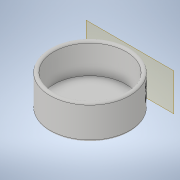
# Autodesk Inventor part: LargeFinderObjectiveCover
Saved by Autodesk Inventor 2021.1 (Build 251245000, 245)
## iProperties
Created: 2018-09-01
Part Number: LargeFinderObjectiveCover
Material: Generic
Document SubType Name: Modeling
Designer: steele
Density: 1 g/cm^3
Appearance: Default
Author: steele
Autodesk Inventor part; units mm, degrees
ref_plane "YZ Plane" through (0, 0, 0) normal (1, 0, 0) x (0, 1, 0)
ref_plane "XZ Plane" through (0, 0, 0) normal (0, 1, 0) x (-1, 0, 0)
sketch "Sketch1" plane through (0, 0, 0) normal (0, 1, 0) x (-1, 0, 0)
  circle A0 centre (0, 0) radius 33.655
  dimension "d0" = 67.31
  constraints: 1 centre point, 1 coincident
  measures "d0" diameter of A0
extrude "Extrusion1" add sketch "Sketch1" along normal blind 3.175
sketch "Sketch2" plane through (0, 3.175, 0) normal (0, 1, 0) x (1, 0, 0)
  circle A0 centre (0, 0) radius 33.655
  circle A1 centre (0, 0) radius 30.48
  dimension "d4" = 60.96
  dimension "d5" = 67.31
  constraints: 2 centre point, 1 coincident
  measures "d4" diameter of A1
  measures "d5" diameter of A0
extrude "Extrusion3" add sketch "Sketch2" along normal blind 25.4
ref_plane "Work Plane1" through (0, 0, -33.655) normal (0, 0, 1) x (1, 0, 0)
sketch "Sketch5" plane through (0, 0, -33.655) normal (0, 0, 1) x (1, 0, 0)
  line L0 (-33.655, 0) -> (-33.655, 28.575) projected
  line L1 (33.655, 0) -> (33.655, 28.575) projected
  line L2 (33.655, 14.2875) -> (-33.655, 14.2875) construction
  line L3 (2.2158, 14.2875) -> (0.248, 14.2875)
  line L4 (0.248, 14.2875) -> (0.248, 13.7688)
  line L5 (0.248, 13.7688) -> (0.8944, 13.7688)
  line L6 (0.8944, 13.7688) -> (0.8944, 9.7262)
  line L7 (0.8944, 9.7262) -> (0.248, 9.7262)
  line L8 (0.248, 9.7262) -> (0.248, 9.2075)
  line L9 (0.248, 9.2075) -> (2.2158, 9.2075)
  line L10 (2.2158, 9.2075) -> (2.2158, 9.7262)
  line L11 (2.2158, 9.7262) -> (1.5695, 9.7262)
  line L12 (1.5695, 9.7262) -> (1.5695, 13.7688)
  line L13 (1.5695, 13.7688) -> (2.2158, 13.7688)
  line L14 (2.2158, 13.7688) -> (2.2158, 14.2875)
  spline S0 degree 2 poles (7.057, 11.7516) (7.057, 12.4473) (6.4931, 13.5671) (6.0196, 13.8799) knots 0 0 0 1 2 2 2
  spline S1 degree 2 poles (6.0196, 13.8799) (5.6327, 14.1228) (4.8381, 14.2875) (4.2206, 14.2875) knots 0 0 0 1 2 2 2
  line L15 (4.2206, 14.2875) -> (3.0515, 14.2875)
  line L16 (3.0515, 14.2875) -> (3.0515, 9.2075)
  line L17 (3.0515, 9.2075) -> (4.2083, 9.2075)
  spline S2 degree 2 poles (4.2083, 9.2075) (4.9246, 9.2075) (5.7397, 9.4216) (6.0279, 9.6109) knots 0 0 0 1 2 2 2
  spline S3 degree 2 poles (6.0279, 9.6109) (6.5178, 9.9362) (7.057, 11.0106) (7.057, 11.7516) knots 0 0 0 1 2 2 2
  spline S4 degree 2 poles (6.3531, 11.7434) (6.3531, 11.1588) (5.9661, 10.3314) (5.5833, 10.0967) knots 0 0 0 1 2 2 2
  spline S5 degree 2 poles (5.5833, 10.0967) (5.3116, 9.9362) (4.6982, 9.7921) (4.2412, 9.7921) knots 0 0 0 1 2 2 2
  line L18 (4.2412, 9.7921) -> (3.7266, 9.7921)
  line L19 (3.7266, 9.7921) -> (3.7266, 13.7029)
  line L20 (3.7266, 13.7029) -> (4.2412, 13.7029)
  spline S6 degree 2 poles (4.2412, 13.7029) (4.6899, 13.7029) (5.3692, 13.5588) (5.645, 13.3654) knots 0 0 0 1 2 2 2
  spline S7 degree 2 poles (5.645, 13.3654) (5.9991, 13.1266) (6.3531, 12.3362) (6.3531, 11.7434) knots 0 0 0 1 2 2 2
  line L21 (13.2815, 14.2875) -> (12.4664, 14.2875)
  line L22 (12.4664, 14.2875) -> (12.4664, 13.316)
  line L23 (12.4664, 13.316) -> (13.2815, 13.316)
  line L24 (13.2815, 13.316) -> (13.2815, 14.2875)
  line L25 (13.2815, 11.447) -> (12.4664, 11.447)
  line L26 (12.4664, 11.447) -> (12.4664, 10.4754)
  line L27 (12.4664, 10.4754) -> (13.2815, 10.4754)
  line L28 (13.2815, 10.4754) -> (13.2815, 11.447)
  line L29 (19.7941, 14.2875) -> (16.6613, 14.2875)
  line L30 (16.6613, 14.2875) -> (16.6613, 13.5671)
  spline S8 degree 2 poles (16.6613, 13.5671) (16.9989, 13.2501) (17.5999, 12.6614) (17.8881, 12.3444) knots 0 0 0 1 2 2 2
  spline S9 degree 2 poles (17.8881, 12.3444) (18.4685, 11.7063) (18.8925, 10.9406) (18.8925, 10.5331) knots 0 0 0 1 2 2 2
  spline S10 degree 2 poles (18.8925, 10.5331) (18.8925, 10.319) (18.7608, 9.9979) (18.6414, 9.895) knots 0 0 0 1 2 2 2
  spline S11 degree 2 poles (18.6414, 9.895) (18.522, 9.7921) (18.2092, 9.6892) (18.0198, 9.6892) knots 0 0 0 1 2 2 2
  spline S12 degree 2 poles (18.0198, 9.6892) (17.8387, 9.6892) (17.4682, 9.7797) (17.2994, 9.8497) knots 0 0 0 1 2 2 2
  spline S13 degree 2 poles (17.2994, 9.8497) (17.1553, 9.9073) (16.8877, 10.072) (16.8054, 10.1296) knots 0 0 0 1 2 2 2
  line L31 (16.8054, 10.1296) -> (16.7683, 10.1296)
  line L32 (16.7683, 10.1296) -> (16.7683, 9.4051)
  spline S14 degree 2 poles (16.7683, 9.4051) (16.9783, 9.3022) (17.7316, 9.1005) (18.0692, 9.1005) knots 0 0 0 1 2 2 2
  spline S15 degree 2 poles (18.0692, 9.1005) (18.7814, 9.1005) (19.5841, 9.8538) (19.5841, 10.496) knots 0 0 0 1 2 2 2
  spline S16 degree 2 poles (19.5841, 10.496) (19.5841, 10.7965) (19.4442, 11.2988) (19.3207, 11.5128) knots 0 0 0 1 2 2 2
  spline S17 degree 2 poles (19.3207, 11.5128) (19.1972, 11.7351) (18.839, 12.1715) (18.6414, 12.3815) knots 0 0 0 1 2 2 2
  spline S18 degree 2 poles (18.6414, 12.3815) (18.3203, 12.7314) (17.534, 13.4806) (17.2994, 13.6988) knots 0 0 0 1 2 2 2
  line L33 (17.2994, 13.6988) -> (19.7941, 13.6988)
  line L34 (19.7941, 13.6988) -> (19.7941, 14.2875)
  line L35 (21.5643, 14.2875) -> (20.7492, 14.2875)
  line L36 (20.7492, 14.2875) -> (20.7492, 13.316)
  line L37 (20.7492, 13.316) -> (21.5643, 13.316)
  line L38 (21.5643, 13.316) -> (21.5643, 14.2875)
  line L39 (25.858, 12.542) -> (25.2528, 12.542)
  line L40 (25.2528, 12.542) -> (25.2528, 14.2875)
  line L41 (25.2528, 14.2875) -> (24.5983, 14.2875)
  line L42 (24.5983, 14.2875) -> (24.5983, 12.542)
  line L43 (24.5983, 12.542) -> (22.3547, 12.542)
  line L44 (22.3547, 12.542) -> (22.3547, 11.8257)
  line L45 (22.3547, 11.8257) -> (24.6271, 9.2075)
  line L46 (24.6271, 9.2075) -> (25.2528, 9.2075)
  line L47 (25.2528, 9.2075) -> (25.2528, 11.9945)
  line L48 (25.2528, 11.9945) -> (25.858, 11.9945)
  line L49 (25.858, 11.9945) -> (25.858, 12.542)
  line L50 (24.5983, 11.9945) -> (24.5983, 10.0103)
  line L51 (24.5983, 10.0103) -> (22.8898, 11.9945)
  line L52 (22.8898, 11.9945) -> (24.5983, 11.9945)
  spline S19 degree 2 poles (29.563, 11.7475) (29.563, 13.1142) (28.7685, 14.3945) (27.941, 14.3945) knots 0 0 0 1 2 2 2
  spline S20 degree 2 poles (27.941, 14.3945) (27.1012, 14.3945) (26.3149, 13.0895) (26.3149, 11.7516) knots 0 0 0 1 2 2 2
  spline S21 degree 2 poles (26.3149, 11.7516) (26.3149, 10.3766) (27.1095, 9.1046) (27.941, 9.1046) knots 0 0 0 1 2 2 2
  spline S22 degree 2 poles (27.941, 9.1046) (28.7767, 9.1046) (29.563, 10.4219) (29.563, 11.7475) knots 0 0 0 1 2 2 2
  spline S23 degree 2 poles (28.6903, 13.2954) (28.7891, 13.0443) (28.8714, 12.2703) (28.8714, 11.7475) knots 0 0 0 1 2 2 2
  spline S24 degree 2 poles (28.8714, 11.7475) (28.8714, 11.2247) (28.7891, 10.4549) (28.6862, 10.1955) knots 0 0 0 1 2 2 2
  spline S25 degree 2 poles (28.6862, 10.1955) (28.5832, 9.9362) (28.2251, 9.6686) (27.941, 9.6686) knots 0 0 0 1 2 2 2
  spline S26 degree 2 poles (27.941, 9.6686) (27.657, 9.6686) (27.2906, 9.9362) (27.1836, 10.2037) knots 0 0 0 1 2 2 2
  spline S27 degree 2 poles (27.1836, 10.2037) (27.0806, 10.4631) (27.0065, 11.2535) (27.0065, 11.7516) knots 0 0 0 1 2 2 2
  spline S28 degree 2 poles (27.0065, 11.7516) (27.0065, 12.2868) (27.0724, 13.0031) (27.1794, 13.283) knots 0 0 0 1 2 2 2
  spline S29 degree 2 poles (27.1794, 13.283) (27.2782, 13.5465) (27.6446, 13.8305) (27.941, 13.8305) knots 0 0 0 1 2 2 2
  spline S30 degree 2 poles (27.941, 13.8305) (28.221, 13.8305) (28.5873, 13.563) (28.6903, 13.2954) knots 0 0 0 1 2 2 2
  spline S31 degree 2 poles (33.3751, 11.7475) (33.3751, 13.1142) (32.5805, 14.3945) (31.7531, 14.3945) knots 0 0 0 1 2 2 2
  spline S32 degree 2 poles (31.7531, 14.3945) (30.9133, 14.3945) (30.127, 13.0895) (30.127, 11.7516) knots 0 0 0 1 2 2 2
  spline S33 degree 2 poles (30.127, 11.7516) (30.127, 10.3766) (30.9215, 9.1046) (31.7531, 9.1046) knots 0 0 0 1 2 2 2
  spline S34 degree 2 poles (31.7531, 9.1046) (32.5888, 9.1046) (33.3751, 10.4219) (33.3751, 11.7475) knots 0 0 0 1 2 2 2
  spline S35 degree 2 poles (32.5023, 13.2954) (32.6011, 13.0443) (32.6835, 12.2703) (32.6835, 11.7475) knots 0 0 0 1 2 2 2
  spline S36 degree 2 poles (32.6835, 11.7475) (32.6835, 11.2247) (32.6011, 10.4549) (32.4982, 10.1955) knots 0 0 0 1 2 2 2
  spline S37 degree 2 poles (32.4982, 10.1955) (32.3953, 9.9362) (32.0371, 9.6686) (31.7531, 9.6686) knots 0 0 0 1 2 2 2
  spline S38 degree 2 poles (31.7531, 9.6686) (31.469, 9.6686) (31.1026, 9.9362) (30.9956, 10.2037) knots 0 0 0 1 2 2 2
  spline S39 degree 2 poles (30.9956, 10.2037) (30.8927, 10.4631) (30.8186, 11.2535) (30.8186, 11.7516) knots 0 0 0 1 2 2 2
  spline S40 degree 2 poles (30.8186, 11.7516) (30.8186, 12.2868) (30.8845, 13.0031) (30.9915, 13.283) knots 0 0 0 1 2 2 2
  spline S41 degree 2 poles (30.9915, 13.283) (31.0903, 13.5465) (31.4567, 13.8305) (31.7531, 13.8305) knots 0 0 0 1 2 2 2
  spline S42 degree 2 poles (31.7531, 13.8305) (32.033, 13.8305) (32.3994, 13.563) (32.5023, 13.2954) knots 0 0 0 1 2 2 2
  spline S43 degree 2 poles (3.8831, 18.1769) (4.1712, 18.5144) (4.4923, 19.5024) (4.4923, 20.1364) knots 0 0 0 1 2 2 2
  spline S44 degree 2 poles (4.4923, 20.1364) (4.4923, 20.7539) (4.1795, 21.7543) (3.8831, 22.0918) knots 0 0 0 1 2 2 2
  spline S45 degree 2 poles (3.8831, 22.0918) (3.5702, 22.4459) (2.7427, 22.7834) (2.2446, 22.7834) knots 0 0 0 1 2 2 2
  spline S46 degree 2 poles (2.2446, 22.7834) (1.73, 22.7834) (0.9067, 22.4335) (0.6062, 22.0918) knots 0 0 0 1 2 2 2
  spline S47 degree 2 poles (0.6062, 22.0918) (0.3139, 21.7543) (0.001, 20.7621) (0.001, 20.1364) knots 0 0 0 1 2 2 2
  spline S48 degree 2 poles (0.001, 20.1364) (0.001, 19.4983) (0.318, 18.5268) (0.6103, 18.1769) knots 0 0 0 1 2 2 2
  spline S49 degree 2 poles (0.6103, 18.1769) (0.9067, 17.8393) (1.7342, 17.4894) (2.2446, 17.4894) knots 0 0 0 1 2 2 2
  spline S50 degree 2 poles (2.2446, 17.4894) (2.7633, 17.4894) (3.5949, 17.8516) (3.8831, 18.1769) knots 0 0 0 1 2 2 2
  spline S51 degree 2 poles (3.7884, 20.1364) (3.7884, 19.6342) (3.5702, 18.8561) (3.3726, 18.6009) knots 0 0 0 1 2 2 2
  spline S52 degree 2 poles (3.3726, 18.6009) (3.1709, 18.3374) (2.6028, 18.0739) (2.2487, 18.0739) knots 0 0 0 1 2 2 2
  spline S53 degree 2 poles (2.2487, 18.0739) (1.8824, 18.0739) (1.3307, 18.3292) (1.1208, 18.6009) knots 0 0 0 1 2 2 2
  spline S54 degree 2 poles (1.1208, 18.6009) (0.9191, 18.8602) (0.705, 19.6424) (0.705, 20.1364) knots 0 0 0 1 2 2 2
  spline S55 degree 2 poles (0.705, 20.1364) (0.705, 21.1368) (1.5448, 22.1989) (2.2487, 22.1989) knots 0 0 0 1 2 2 2
  spline S56 degree 2 poles (2.2487, 22.1989) (2.9527, 22.1989) (3.7884, 21.1368) (3.7884, 20.1364) knots 0 0 0 1 2 2 2
  spline S57 degree 2 poles (9.2389, 20.1405) (9.2389, 20.8362) (8.6749, 21.956) (8.2015, 22.2689) knots 0 0 0 1 2 2 2
  spline S58 degree 2 poles (8.2015, 22.2689) (7.8145, 22.5117) (7.02, 22.6764) (6.4025, 22.6764) knots 0 0 0 1 2 2 2
  line L53 (6.4025, 22.6764) -> (5.2333, 22.6764)
  line L54 (5.2333, 22.6764) -> (5.2333, 17.5964)
  line L55 (5.2333, 17.5964) -> (6.3901, 17.5964)
  spline S59 degree 2 poles (6.3901, 17.5964) (7.1064, 17.5964) (7.9215, 17.8105) (8.2097, 17.9998) knots 0 0 0 1 2 2 2
  spline S60 degree 2 poles (8.2097, 17.9998) (8.6996, 18.3251) (9.2389, 19.3995) (9.2389, 20.1405) knots 0 0 0 1 2 2 2
  spline S61 degree 2 poles (8.5349, 20.1323) (8.5349, 19.5477) (8.148, 18.7203) (7.7651, 18.4856) knots 0 0 0 1 2 2 2
  spline S62 degree 2 poles (7.7651, 18.4856) (7.4934, 18.3251) (6.88, 18.181) (6.4231, 18.181) knots 0 0 0 1 2 2 2
  line L56 (6.4231, 18.181) -> (5.9085, 18.181)
  line L57 (5.9085, 18.181) -> (5.9085, 22.0918)
  line L58 (5.9085, 22.0918) -> (6.4231, 22.0918)
  spline S63 degree 2 poles (6.4231, 22.0918) (6.8718, 22.0918) (7.551, 21.9478) (7.8269, 21.7543) knots 0 0 0 1 2 2 2
  spline S64 degree 2 poles (7.8269, 21.7543) (8.1809, 21.5155) (8.5349, 20.7251) (8.5349, 20.1323) knots 0 0 0 1 2 2 2
  line L59 (13.2815, 22.6764) -> (12.4664, 22.6764)
  line L60 (12.4664, 22.6764) -> (12.4664, 21.7049)
  line L61 (12.4664, 21.7049) -> (13.2815, 21.7049)
  line L62 (13.2815, 21.7049) -> (13.2815, 22.6764)
  line L63 (13.2815, 19.8359) -> (12.4664, 19.8359)
  line L64 (12.4664, 19.8359) -> (12.4664, 18.8643)
  line L65 (12.4664, 18.8643) -> (13.2815, 18.8643)
  line L66 (13.2815, 18.8643) -> (13.2815, 19.8359)
  line L67 (19.7941, 22.6764) -> (16.6613, 22.6764)
  line L68 (16.6613, 22.6764) -> (16.6613, 21.956)
  spline S65 degree 2 poles (16.6613, 21.956) (16.9989, 21.639) (17.5999, 21.0503) (17.8881, 20.7333) knots 0 0 0 1 2 2 2
  spline S66 degree 2 poles (17.8881, 20.7333) (18.4685, 20.0952) (18.8925, 19.3295) (18.8925, 18.922) knots 0 0 0 1 2 2 2
  spline S67 degree 2 poles (18.8925, 18.922) (18.8925, 18.7079) (18.7608, 18.3868) (18.6414, 18.2839) knots 0 0 0 1 2 2 2
  spline S68 degree 2 poles (18.6414, 18.2839) (18.522, 18.181) (18.2092, 18.0781) (18.0198, 18.0781) knots 0 0 0 1 2 2 2
  spline S69 degree 2 poles (18.0198, 18.0781) (17.8387, 18.0781) (17.4682, 18.1686) (17.2994, 18.2386) knots 0 0 0 1 2 2 2
  spline S70 degree 2 poles (17.2994, 18.2386) (17.1553, 18.2962) (16.8877, 18.4609) (16.8054, 18.5185) knots 0 0 0 1 2 2 2
  line L69 (16.8054, 18.5185) -> (16.7683, 18.5185)
  line L70 (16.7683, 18.5185) -> (16.7683, 17.794)
  spline S71 degree 2 poles (16.7683, 17.794) (16.9783, 17.6911) (17.7316, 17.4894) (18.0692, 17.4894) knots 0 0 0 1 2 2 2
  spline S72 degree 2 poles (18.0692, 17.4894) (18.7814, 17.4894) (19.5841, 18.2427) (19.5841, 18.8849) knots 0 0 0 1 2 2 2
  spline S73 degree 2 poles (19.5841, 18.8849) (19.5841, 19.1854) (19.4442, 19.6877) (19.3207, 19.9018) knots 0 0 0 1 2 2 2
  spline S74 degree 2 poles (19.3207, 19.9018) (19.1972, 20.1241) (18.839, 20.5604) (18.6414, 20.7704) knots 0 0 0 1 2 2 2
  spline S75 degree 2 poles (18.6414, 20.7704) (18.3203, 21.1203) (17.534, 21.8695) (17.2994, 22.0877) knots 0 0 0 1 2 2 2
  line L71 (17.2994, 22.0877) -> (19.7941, 22.0877)
  line L72 (19.7941, 22.0877) -> (19.7941, 22.6764)
  line L73 (21.5643, 22.6764) -> (20.7492, 22.6764)
  line L74 (20.7492, 22.6764) -> (20.7492, 21.7049)
  line L75 (20.7492, 21.7049) -> (21.5643, 21.7049)
  line L76 (21.5643, 21.7049) -> (21.5643, 22.6764)
  spline S76 degree 2 poles (25.8003, 21.0297) (25.8003, 21.4208) (25.541, 22.0836) (25.3228, 22.3059) knots 0 0 0 1 2 2 2
  spline S77 degree 2 poles (25.3228, 22.3059) (25.0964, 22.5406) (24.5283, 22.7834) (24.1866, 22.7834) knots 0 0 0 1 2 2 2
  spline S78 degree 2 poles (24.1866, 22.7834) (23.8449, 22.7834) (23.2809, 22.5529) (23.0669, 22.3224) knots 0 0 0 1 2 2 2
  spline S79 degree 2 poles (23.0669, 22.3224) (22.8034, 22.0466) (22.507, 21.1203) (22.507, 20.4452) knots 0 0 0 1 2 2 2
  spline S80 degree 2 poles (22.507, 20.4452) (22.507, 19.7824) (22.7787, 18.7161) (23.0627, 18.3209) knots 0 0 0 1 2 2 2
  spline S81 degree 2 poles (23.0627, 18.3209) (23.3386, 17.934) (24.2113, 17.5017) (24.7835, 17.5017) knots 0 0 0 1 2 2 2
  spline S82 degree 2 poles (24.7835, 17.5017) (24.9523, 17.5017) (25.2487, 17.5347) (25.3599, 17.5717) knots 0 0 0 1 2 2 2
  line L77 (25.3599, 17.5717) -> (25.3599, 18.2263)
  line L78 (25.3599, 18.2263) -> (25.331, 18.2263)
  spline S83 degree 2 poles (25.331, 18.2263) (25.2364, 18.1769) (24.8906, 18.0904) (24.693, 18.0904) knots 0 0 0 1 2 2 2
  spline S84 degree 2 poles (24.693, 18.0904) (24.059, 18.0904) (23.2809, 18.9467) (23.2068, 19.7865) knots 0 0 0 1 2 2 2
  spline S85 degree 2 poles (23.2068, 19.7865) (23.4497, 19.6177) (23.9602, 19.4325) (24.2648, 19.4325) knots 0 0 0 1 2 2 2
  spline S86 degree 2 poles (24.2648, 19.4325) (24.5612, 19.4325) (25.0058, 19.5518) (25.2487, 19.733) knots 0 0 0 1 2 2 2
  spline S87 degree 2 poles (25.2487, 19.733) (25.5286, 19.9429) (25.8003, 20.5934) (25.8003, 21.0297) knots 0 0 0 1 2 2 2
  spline S88 degree 2 poles (25.1087, 21.0585) (25.1087, 20.7457) (24.9441, 20.3217) (24.7629, 20.1735) knots 0 0 0 1 2 2 2
  spline S89 degree 2 poles (24.7629, 20.1735) (24.6271, 20.0664) (24.2895, 19.9964) (24.1125, 19.9964) knots 0 0 0 1 2 2 2
  spline S90 degree 2 poles (24.1125, 19.9964) (23.8737, 19.9964) (23.425, 20.1405) (23.2068, 20.2764) knots 0 0 0 1 2 2 2
  spline S91 degree 2 poles (23.2068, 20.2764) (23.2027, 20.3505) (23.1945, 20.4904) (23.1945, 20.5975) knots 0 0 0 1 2 2 2
  spline S92 degree 2 poles (23.1945, 20.5975) (23.1945, 21.1244) (23.4003, 21.7707) (23.5568, 21.9395) knots 0 0 0 1 2 2 2
  spline S93 degree 2 poles (23.5568, 21.9395) (23.7008, 22.1001) (24.0137, 22.2277) (24.1907, 22.2277) knots 0 0 0 1 2 2 2
  spline S94 degree 2 poles (24.1907, 22.2277) (24.6024, 22.2277) (25.1087, 21.6431) (25.1087, 21.0585) knots 0 0 0 1 2 2 2
  line L79 (29.5342, 22.6764) -> (26.4014, 22.6764)
  line L80 (26.4014, 22.6764) -> (26.4014, 21.956)
  spline S95 degree 2 poles (26.4014, 21.956) (26.739, 21.639) (27.34, 21.0503) (27.6282, 20.7333) knots 0 0 0 1 2 2 2
  spline S96 degree 2 poles (27.6282, 20.7333) (28.2086, 20.0952) (28.6326, 19.3295) (28.6326, 18.922) knots 0 0 0 1 2 2 2
  spline S97 degree 2 poles (28.6326, 18.922) (28.6326, 18.7079) (28.5009, 18.3868) (28.3815, 18.2839) knots 0 0 0 1 2 2 2
  spline S98 degree 2 poles (28.3815, 18.2839) (28.2621, 18.181) (27.9493, 18.0781) (27.7599, 18.0781) knots 0 0 0 1 2 2 2
  spline S99 degree 2 poles (27.7599, 18.0781) (27.5788, 18.0781) (27.2083, 18.1686) (27.0395, 18.2386) knots 0 0 0 1 2 2 2
  spline S100 degree 2 poles (27.0395, 18.2386) (26.8954, 18.2962) (26.6278, 18.4609) (26.5455, 18.5185) knots 0 0 0 1 2 2 2
  line L81 (26.5455, 18.5185) -> (26.5084, 18.5185)
  line L82 (26.5084, 18.5185) -> (26.5084, 17.794)
  spline S101 degree 2 poles (26.5084, 17.794) (26.7184, 17.6911) (27.4717, 17.4894) (27.8093, 17.4894) knots 0 0 0 1 2 2 2
  spline S102 degree 2 poles (27.8093, 17.4894) (28.5215, 17.4894) (29.3242, 18.2427) (29.3242, 18.8849) knots 0 0 0 1 2 2 2
  spline S103 degree 2 poles (29.3242, 18.8849) (29.3242, 19.1854) (29.1843, 19.6877) (29.0608, 19.9018) knots 0 0 0 1 2 2 2
  spline S104 degree 2 poles (29.0608, 19.9018) (28.9373, 20.1241) (28.5791, 20.5604) (28.3815, 20.7704) knots 0 0 0 1 2 2 2
  spline S105 degree 2 poles (28.3815, 20.7704) (28.0604, 21.1203) (27.2741, 21.8695) (27.0395, 22.0877) knots 0 0 0 1 2 2 2
  line L83 (27.0395, 22.0877) -> (29.5342, 22.0877)
  line L84 (29.5342, 22.0877) -> (29.5342, 22.6764)
  spline S106 degree 2 poles (33.2927, 21.0627) (33.2927, 21.429) (33.0581, 22.0548) (32.844, 22.2853) knots 0 0 0 1 2 2 2
  spline S107 degree 2 poles (32.844, 22.2853) (32.6299, 22.5159) (31.9919, 22.7834) (31.5967, 22.7834) knots 0 0 0 1 2 2 2
  spline S108 degree 2 poles (31.5967, 22.7834) (31.2344, 22.7834) (30.5263, 22.6229) (30.267, 22.4953) knots 0 0 0 1 2 2 2
  line L85 (30.267, 22.4953) -> (30.267, 21.7748)
  line L86 (30.267, 21.7748) -> (30.3164, 21.7748)
  spline S109 degree 2 poles (30.3164, 21.7748) (30.3946, 21.8325) (30.6869, 21.9807) (30.8639, 22.0466) knots 0 0 0 1 2 2 2
  spline S110 degree 2 poles (30.8639, 22.0466) (31.0656, 22.1165) (31.3991, 22.1948) (31.609, 22.1948) knots 0 0 0 1 2 2 2
  spline S111 degree 2 poles (31.609, 22.1948) (31.8148, 22.1948) (32.2018, 22.0466) (32.3418, 21.886) knots 0 0 0 1 2 2 2
  spline S112 degree 2 poles (32.3418, 21.886) (32.4694, 21.7337) (32.6011, 21.3302) (32.6011, 21.0585) knots 0 0 0 1 2 2 2
  spline S113 degree 2 poles (32.6011, 21.0585) (32.6011, 20.7868) (32.4529, 20.441) (32.313, 20.3258) knots 0 0 0 1 2 2 2
  spline S114 degree 2 poles (32.313, 20.3258) (32.1689, 20.1982) (31.7407, 20.0911) (31.4814, 20.0911) knots 0 0 0 1 2 2 2
  spline S115 degree 2 poles (31.4814, 20.0911) (31.2015, 20.0911) (30.6457, 20.1776) (30.4769, 20.2146) knots 0 0 0 1 2 2 2
  line L87 (30.4769, 20.2146) -> (30.4769, 17.5964)
  line L88 (30.4769, 17.5964) -> (33.2639, 17.5964)
  line L89 (33.2639, 17.5964) -> (33.2639, 18.1933)
  line L90 (33.2639, 18.1933) -> (31.1315, 18.1933)
  line L91 (31.1315, 18.1933) -> (31.1315, 19.5477)
  spline S116 degree 2 poles (31.1315, 19.5477) (31.255, 19.5313) (31.4937, 19.5189) (31.5925, 19.5189) knots 0 0 0 1 2 2 2
  spline S117 degree 2 poles (31.5925, 19.5189) (31.9836, 19.5189) (32.5229, 19.6465) (32.7699, 19.8359) knots 0 0 0 1 2 2 2
  spline S118 degree 2 poles (32.7699, 19.8359) (33.021, 20.0253) (33.2927, 20.6016) (33.2927, 21.0627) knots 0 0 0 1 2 2 2
  point P0 (0, 0)
  constraints: 2 end point, 2 midpoint, 1 horizontal
emboss "Emboss1" sketch "Sketch5" operation cut depth 1.27 direction (0, 0, -1) wrap yes faces at (-33.2192, 10.5833, -5.3986)
fillet "Fillet1" radius 1.5875 2 edges at (-33.655, 28.575, 0) (-30.48, 28.575, 0)
fillet "Fillet2" radius 1.5875 1 edges at (33.655, 0, 0)
equation "\"d0\" = lensCoverOD"
equation "\"d2\" = wallThickness"
equation "\"d4\" = lensCoverID"
equation "\"d5\" = lensCoverOD"
equation "\"d9\" = lensCoverLength"
equation "\"d11\" = textDepth"
equation "\"d13\" = filetRadius"
equation "\"d14\" = filetRadius"
equation "\"objectiveOD\" = 60.325"
equation "\"lensCoverLength\" = 25.4"
equation "\"wallThickness\" = 3.175"
equation "\"lensCoverOD\" = lensCoverID + 2 * wallThickness"
equation "\"clearance\" = 0.635"
equation "\"lensCoverID\" = objectiveOD + clearance"
equation "\"textDepth\" = 1.27"
equation "\"filetRadius\" = 1.5875"
body "Solid1"
